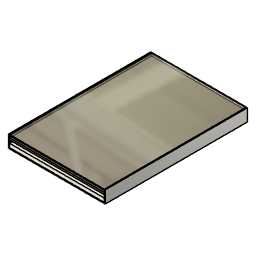
Solar Collector v2 (Autodesk Fusion 360 design; units mm, degrees)
Autodesk Fusion 360 part; units mm, degrees
sketch "Sketch1" plane through (0, 0, 0) normal (0, 0, 1) x (1, 0, 0)
  line L0 (0, 0) -> (1000, 0)
  line L1 (1000, 0) -> (1000, 40)
  line L2 (1000, 40) -> (0, 40)
  line L3 (0, 40) -> (0, 0)
  line L4 (0, 90) -> (1000, 90)
  line L5 (1000, 90) -> (1000, 70)
  line L6 (1000, 70) -> (0, 70)
  line L7 (0, 70) -> (0, 90)
  line L8 (0, 120) -> (1000, 120)
  line L9 (1000, 120) -> (1000, 110)
  line L10 (1000, 110) -> (0, 110)
  line L11 (0, 110) -> (0, 120)
  line L12 (0, 120) -> (-10, 120)
  line L13 (-10, 120) -> (-10, -10)
  line L14 (-10, -10) -> (1000, -10)
  line L15 (1000, -10) -> (1010, -10)
  line L16 (1010, -10) -> (1010, 120)
  line L17 (1010, 120) -> (1000, 120)
  line L18 (1000, 0) -> (1000, 120)
  line L19 (0, 120) -> (0, 0)
  dimension "d1" = 1000
  dimension "d2" = 40
  dimension "d3" = 1000
  dimension "d4" = 20
  dimension "d5" = 1000
  dimension "d6" = 10
  dimension "d7" = 10
  dimension "d8" = 1010
  constraint horizontal L0
  constraint vertical L1
  constraint horizontal L2
  constraint vertical L3
  constraint coincident L0.start L3.end
  constraint horizontal L4
  constraint vertical L5
  constraint horizontal L6
  constraint vertical L7
  constraint horizontal L8
  constraint vertical L9
  constraint horizontal L10
  constraint vertical L11
  constraint perpendicular L11 L12
  constraint perpendicular L8 L13
  constraint perpendicular L13 L14
  constraint perpendicular L1 L15
  constraint perpendicular L2 L16
  constraint parallel L9 L18
  measures "d1" distance of L0.start L0.end
  measures "d2" distance of L0.start L2.end
  measures "d3" distance of L4.start L4.end
  measures "d4" distance of L4.start L6.end
  measures "d5" distance of L8.start L8.end
  measures "d6" distance of L8.start L10.end
  measures "d7" distance of L8.start L12.end
  measures "d8" distance of L13.end L14.end
sketch "Sketch2" plane through (0, 0, 0) normal (0, 0, 1) x (1, 0, 0)
  line L0 (0, 0) -> (1000, 0)
  line L1 (1000, 0) -> (1000, 40)
  line L2 (1000, 40) -> (0, 40)
  line L3 (0, 40) -> (0, 0)
  dimension "d11" = 1000
  dimension "d12" = 40
  constraint horizontal L0
  constraint vertical L1
  constraint horizontal L2
  constraint vertical L3
  constraint coincident L0.start L3.end
  measures "d11" distance of L0.start L0.end
  measures "d12" distance of L0.start L2.end
sketch "Sketch3" plane through (0, 0, 0) normal (0, 0, 1) x (1, 0, 0)
  line L0 (0, 70) -> (1000, 70)
  line L1 (1000, 70) -> (1000, 90)
  line L2 (1000, 90) -> (0, 90)
  line L3 (0, 90) -> (0, 70)
  dimension "d15" = 1000
  dimension "d16" = 20
  constraint horizontal L0
  constraint vertical L1
  constraint horizontal L2
  constraint vertical L3
  measures "d15" distance of L0.start L0.end
  measures "d16" distance of L0.start L2.end
sketch "Sketch4" plane through (0, 0, 1400) normal (0, 0, 1) x (1, 0, 0)
  line L0 (0, 40) -> (0, 0)
  line L1 (0, 0) -> (1000, 0)
  line L2 (1000, 0) -> (1000, 40)
  line L3 (1000, 40) -> (0, 40)
  line L4 (0, 120) -> (1000, 120)
  line L5 (1000, 120) -> (1000, 110)
  line L6 (1000, 110) -> (0, 110)
  line L7 (0, 110) -> (0, 120)
  dimension "d19" = 1000
  dimension "d20" = 10
  constraint horizontal L4
  constraint vertical L5
  constraint horizontal L6
  constraint vertical L7
  measures "d19" distance of L4.start L4.end
  measures "d20" distance of L4.start L6.end
extrude "Extrude5" add sketch "Sketch1" along normal blind 1500 contours L0 L1 L3 L5 L7 L9 L11 L12 L13 L14 L15 L16 L17 L18 L19 makes body 1
extrude "Extrude6" add sketch "Sketch2" along normal blind 1500 separate body makes body 2
extrude "Extrude7" add sketch "Sketch3" along normal blind 1500 separate body makes body 3
extrude "Extrude8" add sketch "Sketch4" along normal blind 100 and the other way blind 1400 separate body contours L4 L5 L6 L7 makes body 4
